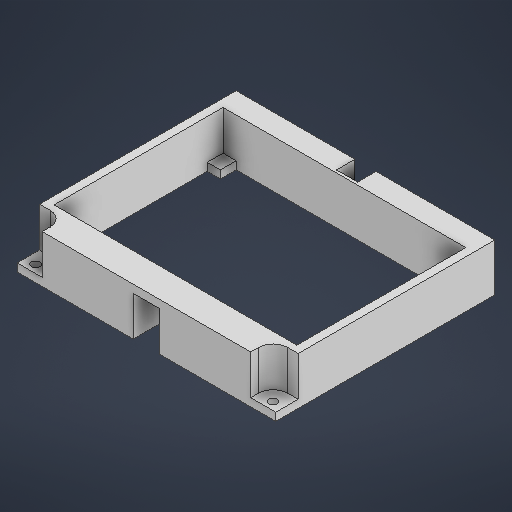
# Autodesk Inventor part: Część4
Saved by Autodesk Inventor 2026 (Build 300175000, 175)
## iProperties
Created: 2026-05-09
Part Number: Część4
Material: Ogólny
Document SubType Name: Modeling
Designer: Patryk Lombardo
Density: 1 g/cm^3
Appearance: Domyślna
Author: Patryk Lombardo
Autodesk Inventor part; units mm, degrees
ref_plane "YZ Plane" through (0, 0, 0) normal (1, 0, 0) x (0, 1, 0)
ref_plane "XZ Plane" through (0, 0, 0) normal (0, 1, 0) x (-1, 0, 0)
ref_plane "XY Plane" through (0, 0, 0) normal (0, 0, 1) x (1, 0, 0)
sketch "Szkic1" plane through (0, 0, 0) normal (0, 1, 0) x (-1, 0, 0)
  line L0 (0, 0) -> (-98, 0)
  line L1 (-98, 0) -> (-98, -83)
  line L2 (-98, -83) -> (0, -83)
  line L3 (0, -83) -> (0, 0)
  line L4 (-3, -11) -> (-95, -11)
  line L5 (-95, -11) -> (-95, -75)
  line L6 (-95, -75) -> (-3, -75)
  line L7 (-3, -75) -> (-3, -11)
  dimension "d0" = 83
  dimension "d1" = 98
  dimension "d2" = 92
  dimension "d3" = 3
  dimension "d4" = 8
  dimension "d5" = 64
  constraints: 16 end point, 4 parallel, 2 horizontal, 2 perpendicular
  measures "d0" distance of L0.end L1.end
  measures "d1" distance of L1.end L2.end
  measures "d2" distance of L5.end L6.end
  measures "d3" distance between parallel lines of L1 L5
  measures "d4" distance between parallel lines of L2 L6
  measures "d5" distance of L4.end L5.end
extrude "Wyciągnięcie proste1" add sketch "Szkic1" along normal blind 18
sketch "Szkic2" plane through (0, 0, 0) normal (0, 0, 1) x (1, 0, 0)
  line L0 (0, 0) -> (49, 0) construction
  line L1 (49, 0) -> (49, 15) construction
  line L2 (44, 15) -> (54, 15)
  line L3 (44, 15) -> (44, 0)
  line L4 (44, 0) -> (54, 0)
  line L5 (54, 0) -> (54, 15)
  dimension "d8" = 15
  dimension "d9" = 49
  dimension "d64" = 10
  constraints: 12 end point, 3 horizontal, 3 perpendicular, 1 midpoint, 1 point on line
  measures "d8" distance of L0.end L1.end
  measures "d9" distance of L0.start L0.end
  measures "d64" distance of L2.start L2.end
sketch "Szkic3" plane through (0, 18, 0) normal (0, 1, 0) x (1, 0, 0)
  line L0 (0, 0) -> (0, 83) construction
  line L1 (0, 83) -> (49, 83) construction
  line L2 (49, 83) -> (49, 80) construction
  line L3 (49, 80) -> (49, 76) construction
  circle A0 centre (49, 80) radius 1.6
  line L4 (45, 76) -> (53, 76)
  line L5 (45, 76) -> (45, 83)
  line L6 (53, 76) -> (53, 83)
  line L7 (53, 83) -> (45, 83)
  dimension "d20" = 3
  dimension "d21" = 4
  dimension "d22" = 49
  dimension "d23" = 83
  dimension "d24" = 3.2
  dimension "d25" = 8
  constraints: 16 end point, 4 perpendicular, 2 point on line, 2 vertical, 1 centre point, 1 coincident, 1 horizontal, 1 midpoint
  measures "d20" distance of L1.end L2.end
  measures "d21" distance of L2.end L3.end
  measures "d22" distance of L0.end L1.end
  measures "d23" distance of L0.start L0.end
  measures "d24" diameter of A0
  measures "d25" distance of L4.start L4.end
extrude "Wyciągnięcie proste3" cut sketch "Szkic3" against normal blind 15 contours A0 | L5 L7 L6 L4
extrude "Wyciągnięcie proste4" cut sketch "Szkic3" against normal through all contours A0
sketch "Szkic4" plane through (0, 18, 0) normal (0, 1, 0) x (1, 0, 0)
  line L0 (0, 0) -> (0, 3)
  line L1 (0, 3) -> (4, 3)
  circle A0 centre (4, 3) radius 1.6
  circle A1 centre (4, 3) radius 5.5
  line L2 (9.5, 3) -> (9.5, -5)
  line L3 (4, 8.5) -> (-4, 8.5)
  line L4 (-4, 8.5) -> (-4, -5)
  line L5 (-4, -5) -> (9.5, -5)
  line L6 (0, 0) -> (98, 0) construction
  line L7 (98, 0) -> (98, 3) construction
  line L8 (98, 3) -> (94, 3) construction
  circle A2 centre (94, 3) radius 1.6
  circle A3 centre (94, 3) radius 5.5
  line L9 (94, 8.5) -> (102, 8.5)
  line L10 (102, 8.5) -> (102, -5)
  line L11 (102, -5) -> (88.5, -5)
  line L12 (88.5, -5) -> (88.5, 3)
  dimension "d30" = 4
  dimension "d31" = 3
  dimension "d32" = 3.2
  dimension "d33" = 11
  dimension "d34" = 8
  dimension "d35" = 8
  dimension "d36" = 98
  dimension "d37" = 3
  dimension "d38" = 4
  dimension "d39" = 11
  dimension "d40" = 3.2
  dimension "d41" = 8
  dimension "d42" = 8
  constraints: 26 end point, 6 perpendicular, 4 centre point, 4 coincident, 4 point on circle, 4 tangent, 3 horizontal, 3 vertical, 1 parallel
  measures "d30" distance of L0.end L1.end
  measures "d31" distance of L0.start L0.end
  measures "d32" diameter of A0
  measures "d33" diameter of A1
  measures "d34" distance of L2.start L2.end
  measures "d35" distance of L3.start L3.end
  measures "d36" distance of L0.start L6.end
  measures "d37" distance of L6.end L7.end
  measures "d38" distance of L7.end L8.end
  measures "d39" diameter of A3
  measures "d40" diameter of A2
  measures "d41" distance of L9.start L9.end
  measures "d42" distance of L11.end L12.end
extrude "Wyciągnięcie proste5" cut sketch "Szkic4" against normal blind 15 contours A0 | A1 | L2 L5 L4 L3 A1 | A2 | A3 | A3 L9 L10 L11 L12
extrude "Wyciągnięcie proste6" cut sketch "Szkic4" against normal through all contours A0 | A2
sketch "Szkic5" plane through (0, 0, 0) normal (0, -1, 0) x (1, 0, 0)
  line L0 (0, 0) -> (0, -11) construction
  line L1 (0, -11) -> (0, -75) construction
  line L2 (0, -75) -> (3, -75) construction
  line L3 (0, -11) -> (3, -11) construction
  line L4 (0, 0) -> (98, 0) construction
  line L5 (98, 0) -> (98, -11) construction
  line L6 (98, -11) -> (95, -11) construction
  line L7 (98, -11) -> (98, -75) construction
  line L8 (98, -75) -> (95, -75) construction
  line L9 (3, -11) -> (8, -11)
  line L10 (8, -11) -> (8, -22)
  line L11 (8, -22) -> (3, -22)
  line L12 (3, -22) -> (3, -11)
  line L13 (3, -75) -> (8, -75)
  line L14 (8, -75) -> (8, -69)
  line L15 (8, -69) -> (3, -69)
  line L16 (3, -69) -> (3, -75)
  line L17 (95, -11) -> (90, -11)
  line L18 (90, -11) -> (90, -22)
  line L19 (90, -22) -> (95, -22)
  line L20 (95, -22) -> (95, -11)
  line L21 (95, -75) -> (90, -75)
  line L22 (90, -75) -> (90, -69)
  line L23 (90, -69) -> (95, -69)
  line L24 (95, -69) -> (95, -75)
  dimension "d47" = 3
  dimension "d48" = 3
  dimension "d49" = 11
  dimension "d50" = 64
  dimension "d51" = 98
  dimension "d52" = 11
  dimension "d53" = 3
  dimension "d54" = 3
  dimension "d55" = 64
  dimension "d56" = 11
  dimension "d57" = 5
  dimension "d58" = 6
  dimension "d59" = 5
  dimension "d60" = 6
  dimension "d61" = 11
  constraints: 50 end point, 8 parallel, 8 perpendicular, 6 horizontal, 3 point on line, 2 vertical
  measures "d47" distance of L0.end L3.end
  measures "d48" distance of L1.end L2.end
  measures "d49" distance of L0.start L0.end
  measures "d50" distance of L0.end L1.end
  measures "d51" distance of L0.start L4.end
  measures "d52" distance of L4.end L5.end
  measures "d53" distance of L5.end L6.end
  measures "d54" distance of L7.end L8.end
  measures "d55" distance of L5.end L7.end
  measures "d56" distance of L17.end L18.end
  measures "d57" distance of L6.end L17.end
  measures "d58" distance of L21.end L22.end
  measures "d59" distance of L14.end L15.end
  measures "d60" distance of L13.end L14.end
  measures "d61" distance of L9.end L10.end
extrude "Wyciągnięcie proste7" add sketch "Szkic5" against normal blind 3
extrude "Wyciągnięcie proste8" cut sketch "Szkic2" against normal blind 15
